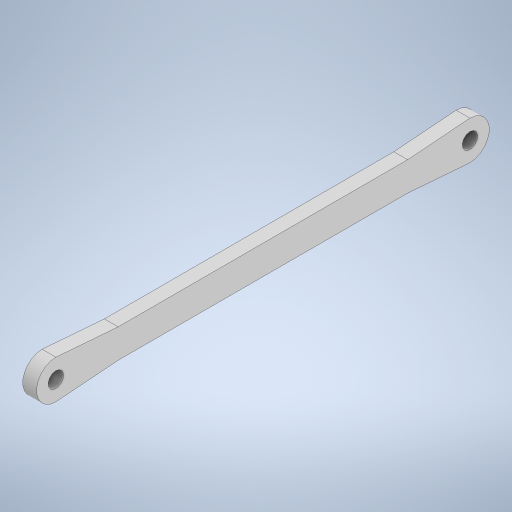
# Autodesk Inventor part: Bielette
Saved by Autodesk Inventor 2023 (Build 270158000, 158)
## iProperties
Created: 2023-03-06
Part Number: Bielette
Material: Générique
Document SubType Name: Modeling
Designer: pined
Density: 1 g/cm^3
Appearance: Par défaut
Author: pined
Autodesk Inventor part; units mm, degrees
ref_plane "YZ Plane" through (0, 0, 0) normal (1, 0, 0) x (0, 1, 0)
ref_plane "XZ Plane" through (0, 0, 0) normal (0, 1, 0) x (-1, 0, 0)
ref_plane "XY Plane" through (0, 0, 0) normal (0, 0, 1) x (1, 0, 0)
sketch "Esquisse1" plane through (0, 0, 0) normal (1, 0, 0) x (0, 1, 0)
  circle A0 centre (-0.2961, 130.2069) radius 2.8
  circle A1 centre (-0.2961, -19.7931) radius 2.8
  circle A2 centre (-0.2961, 130.2069) radius 7
  circle A3 centre (-0.2961, -19.7931) radius 7
  line L0 (4.9445, 125.5662) -> (-5.5366, 125.5662)
  line L1 (-5.5366, 125.5662) -> (-5.5366, -15.1524)
  line L2 (-5.5366, -15.1524) -> (4.9445, -15.1524)
  line L3 (4.9445, -15.1524) -> (4.9445, 125.5662)
  line L4 (6.7039, 130.2069) -> (4.9445, 107.6407)
  line L5 (-0.2961, 125.5662) -> (-0.2961, -15.1524)
  line L6 (-7.2961, 130.2069) -> (-5.5366, 107.6407)
  line L7 (-5.5366, 55.2069) -> (4.9445, 55.2069)
  line L8 (6.7039, -19.7931) -> (4.9445, 2.7731)
  line L9 (-7.2961, -19.7931) -> (-5.5366, 2.7731)
  point P0 (0, 0)
  point P1 (6.7039, -19.7931)
  dimension "d3" = 14
  dimension "d0" = 5.6
  dimension "d1" = 5.6
  dimension "d2" = 150
  dimension "d4" = 14
  constraints: 20 end point, 6 symmetric about line, 4 midpoint, 3 centre point, 3 point on circle, 2 coincident, 2 parallel, 1 horizontal, 1 perpendicular, 1 point on line, 3 other
  measures "d0" diameter of A0
  measures "d1" diameter of A1
  measures "d2" distance of A1.centre A0.centre
  measures "d4" diameter of A2
extrude "Extrusion1" add sketch "Esquisse1" along normal blind 5 contours L4 A2 L0 L6 | L4 L3 A2 | A2 L1 L6 | L3 L7 L5 A2 | A2 L5 L0 | L0 L5 A2 | A2 L5 L7 L1 | L3 A3 L5 L7 | L7 L5 A3 L1 | L8 A3 L3 | L1 A3 L9 | L5 L2 A3 | A3 L2 L5 | A3 L8 L9 L2
